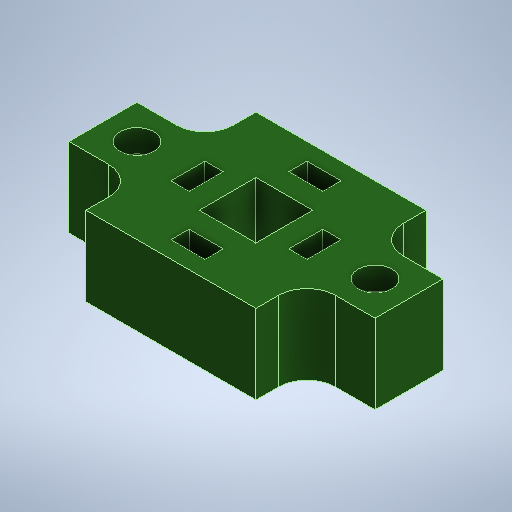
# Autodesk Inventor part: Lower Path Fixation
Saved by Autodesk Inventor 2025.4 (Build 294407000, 407)
## iProperties
Created: 2026-04-10
Part Number: Lower Path Fixation
Material: Generic
Document SubType Name: Modeling
Designer: lenovo
Density: 1 g/cm^3
Appearance: Default(1)
Author: lenovo
Autodesk Inventor part; units mm, degrees
ref_plane "YZ Plane" through (0, 0, 0) normal (1, 0, 0) x (0, 1, 0)
ref_plane "XZ Plane" through (0, 0, 0) normal (0, 1, 0) x (-1, 0, 0)
ref_plane "XY Plane" through (0, 0, 0) normal (0, 0, 1) x (1, 0, 0)
sketch "Sketch2" plane through (0, 0, 0) normal (0, 1, 0) x (-1, 0, 0)
  line L0 (-15, 15) -> (15, 15)
  line L1 (15, 15) -> (15, -15)
  line L2 (15, -15) -> (-15, -15)
  line L3 (-15, -15) -> (-15, 15)
  line L4 (-15, 15) -> (15, -15) construction
  line L5 (15, 15) -> (-15, -15) construction
  line L6 (15, 6) -> (27, 6)
  line L7 (27, 6) -> (27, -6)
  line L8 (27, -6) -> (15, -6)
  line L9 (15, -6) -> (15, 6)
  line L10 (0, 15) -> (0, -15)
  line L11 (-15, 6) -> (-27, 6)
  line L12 (-27, 6) -> (-27, -6)
  line L13 (-27, -6) -> (-15, -6)
  line L14 (-15, -6) -> (-15, 6)
  circle A0 centre (21, 0) radius 1.6
  circle A1 centre (-21, 0) radius 1.6
  point P0 (0, 0)
  point P1 (15, 0)
  point P2 (-15, 0)
  point P3 (21, 6)
  point P4 (0, 0)
  dimension "d2" = 30
  dimension "d16" = 12
  dimension "d17" = 3.2
  constraints: 30 end point, 8 midpoint, 6 symmetric about line, 4 parallel, 4 perpendicular, 2 centre point, 2 horizontal, 1 horizontal alignment, 1 vertical alignment, 1 other
  measures "d2" distance of L1.end L2.end
  measures "d16" distance of L6.end L7.end
  measures "d17" diameter of A0
extrude "Extrusion1" add sketch "Sketch2" along normal blind 14
sketch "Sketch3" plane through (0, 14, 0) normal (0, 1, 0) x (1, 0, 0)
  line L0 (-3, -12) -> (3, -12)
  line L1 (3, -12) -> (3, -8.8)
  line L2 (3, -8.8) -> (-3, -8.8)
  line L3 (-3, -8.8) -> (-3, -12)
  line L4 (-3, -12) -> (3, -8.8) construction
  line L5 (3, -12) -> (-3, -8.8) construction
  line L6 (-15, 15) -> (-15, -15) projected
  line L7 (-15, 0) -> (15, 0)
  line L8 (15, -15) -> (15, 15) projected
  line L9 (-12, -3) -> (-8.8, -3)
  line L10 (-8.8, -3) -> (-8.8, 3)
  line L11 (-8.8, 3) -> (-12, 3)
  line L12 (-12, 3) -> (-12, -3)
  line L13 (-12, -3) -> (-8.8, 3) construction
  line L14 (-8.8, -3) -> (-12, 3) construction
  line L15 (-15, -15) -> (15, -15) projected
  line L16 (0, -15) -> (0, 15)
  line L17 (15, 15) -> (-15, 15) projected
  line L18 (-3, 12) -> (3, 12)
  line L19 (3, 12) -> (3, 8.8)
  line L20 (3, 8.8) -> (-3, 8.8)
  line L21 (-3, 8.8) -> (-3, 12)
  line L22 (12, -3) -> (8.8, -3)
  line L23 (8.8, -3) -> (8.8, 3)
  line L24 (8.8, 3) -> (12, 3)
  line L25 (12, 3) -> (12, -3)
  line L26 (12, -3) -> (8.8, 3) construction
  line L27 (8.8, -3) -> (12, 3) construction
  point P0 (0, 0)
  point P1 (0, -10.4)
  point P2 (-10.4, 0)
  point P3 (0, 0)
  point P4 (10.4, 0)
  dimension "d10" = 3
  dimension "d11" = 3
  dimension "d12" = 6
  dimension "d13" = 3.2
  constraints: 48 end point, 9 midpoint, 9 symmetric about line, 4 parallel, 4 perpendicular, 2 horizontal, 1 point on line, 1 vertical alignment
  measures "d10" distance between parallel lines of L15 L0
  measures "d11" distance between parallel lines of L6 L12
  measures "d12" distance of L0.start L0.end
  measures "d13" distance of L0.end L1.end
extrude "Extrusion2" cut sketch "Sketch3" against normal through all contours L3 L2 L16 L0 | L16 L2 L1 L0 | L10 L9 L12 L7 | L7 L12 L11 L10 | L23 L24 L25 L7 | L7 L25 L22 L23 | L20 L21 L18 L16 | L16 L18 L19 L20
sketch "Sketch4" plane through (0, 14, 0) normal (0, 1, 0) x (1, 0, 0)
  circle A0 centre (-21, 0) radius 3
  circle A1 centre (-21, 0) radius 1.6 projected
  line L0 (-15, -15) -> (15, -15) projected
  line L1 (0, -15) -> (0, 15)
  line L2 (15, 15) -> (-15, 15) projected
  circle A2 centre (21, 0) radius 3
  point P0 (0, 0)
  dimension "d18" = 6
  constraints: 2 centre point, 2 end point, 2 midpoint, 1 concentric, 1 symmetric about line, 1 other
  measures "d18" diameter of A0
extrude "Extrusion3" cut sketch "Sketch4" against normal blind 4 contours A0 | A1 | A2
fillet "Fillet1" radius 5 4 edges at (15, 7, -6) (15, 7, 6) (-15, 7, 6) (-15, 7, -6)
sketch "Sketch5" plane through (0, 14, 0) normal (0, 1, 0) x (1, 0, 0)
  line L0 (5, 5) -> (-5, 5)
  line L1 (-5, 5) -> (-5, -5)
  line L2 (-5, -5) -> (5, -5)
  line L3 (5, -5) -> (5, 5)
  line L4 (5, 5) -> (-5, -5) construction
  line L5 (-5, 5) -> (5, -5) construction
  point P0 (0, 0)
  dimension "d22" = 10
  constraints: 12 end point, 2 midpoint, 2 parallel, 2 perpendicular, 1 horizontal
  measures "d22" distance of L2.end L1.end
extrude "Extrusion4" cut sketch "Sketch5" against normal through all
equation "\"d11\" = d10"
body "Solid1"
